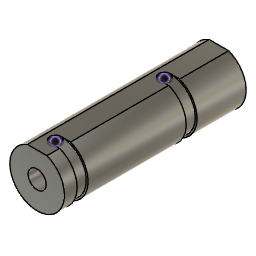
Chronograph v3 (Autodesk Fusion 360 design; units mm, degrees)
Autodesk Fusion 360 part; units mm, degrees
sketch "Sketch1" plane through (0, 0, 0) normal (0, 1, 0) x (1, 0, 0)
  circle A0 centre (0, 0) radius 7.25
  circle A1 centre (0, 0) radius 2.25
  dimension "d1" = 14.5
  dimension "d2" = 4.5
  constraint coincident A0.centre A1.centre
  measures "d1" diameter of A0
  measures "d2" diameter of A1
extrude "Extrude1" add sketch "Sketch1" along normal blind 20 makes body 1
sketch "Sketch2" plane through (0, 0, 0) normal (0, -1, 0) x (1, 0, 0)
  circle A0 centre (0, 0) radius 2.25
  circle A1 centre (0, 0) radius 7.25
  circle A2 centre (0, 0) radius 7.25
  circle A3 centre (0, 0) radius 7.35
  circle A4 centre (0, 0) radius 15
  circle A5 centre (0, 0) radius 5
  dimension "d5" = 0.1
  dimension "d6" = 30
  dimension "d7" = 10
  constraint concentric A2 A4
  constraint coincident A0.centre A1.centre
  measures "d6" diameter of A4
  measures "d7" diameter of A5
extrude "Extrude2" add sketch "Sketch2" against normal blind 20 separate body contours A4 makes body 2
extrude "Extrude3" add sketch "Sketch2" along normal blind 80 contours A1 A2 | A3 | A4 bodies 2
sketch "Sketch3" plane through (0, 0, 0) normal (0, 0, 1) x (1, 0, 0)
  line L0 (-27.4717, -70) -> (30.3284, -70) construction
  line L1 (-28.0905, -10) -> (-26.9766, -10)
  line L2 (-26.9766, -10) -> (39.3636, -10) construction
  line L3 (-15, -80) -> (15, -80)
  circle A0 through (-15, -80, 0) (7.5, -80, 12.9904) (7.5, -80, -12.9904)
  line L4 (0, -70) -> (0, -10) construction
  circle A1 centre (0, -10) radius 2.5
  circle A2 centre (0, -70) radius 2.5
  dimension "d12" = 10
  dimension "d13" = 60
  dimension "d14" = 5
  dimension "d15" = 5
  constraint horizontal L0
  constraint horizontal L1
  constraint parallel L1 L2
  constraint coincident L2 L4.end
  constraint coincident L0 L4.start
  constraint coincident L4.end A1.centre
  constraint coincident L4.start A2.centre
  measures "d12" distance of L0 L3
  measures "d13" distance of L0 L2
  measures "d14" diameter of A1
  measures "d15" diameter of A2
extrude "Extrude4" cut sketch "Sketch3" along normal mid plane 32 bodies 2
ref_plane "WorkPlane1" through (0, 0, 13) normal (0, 0, 1) x (1, 0, 0)
ref_plane "WorkPlane2" through (0, 0, -13) normal (0, 0, 1) x (1, 0, 0)
sketch "Sketch4" plane through (0, 0, 13) normal (0, 0, 1) x (1, 0, 0)
  circle A0 centre (0, -10) radius 2.5
  circle A1 centre (0, -10) radius 3
  circle A2 centre (0, -70) radius 2.5
  circle A3 centre (0, -70) radius 3
  dimension "d20" = 6
  dimension "d21" = 6
  constraint concentric A0 A1
  constraint concentric A2 A3
  measures "d20" diameter of A1
  measures "d21" diameter of A3
extrude "Extrude5" cut sketch "Sketch4" along normal blind 9 contours A0 | A1 | A2 | A3 bodies 2
sketch "Sketch5" plane through (0, 0, -13) normal (0, 0, 1) x (1, 0, 0)
  circle A0 centre (0, -10) radius 3
  circle A1 centre (0, -70) radius 3
extrude "Extrude6" cut sketch "Sketch5" against normal blind 6 bodies 2
ref_plane "WorkPlane3" through (0, -70, 14) normal (0, 0, 1) x (1, 0, 0)
sketch "Sketch6" plane through (0, 0, 14) normal (0, 0, 1) x (1, 0, 0)
  line L0 (-34.0055, 38.0437) -> (36.5157, 38.0437)
  line L1 (36.5157, 38.0437) -> (36.5157, -94.6762)
  line L2 (36.5157, -94.6762) -> (-34.0055, -94.6762)
  line L3 (-34.0055, -94.6762) -> (-34.0055, 38.0437)
  constraint horizontal L0
  constraint vertical L1
  constraint horizontal L2
  constraint vertical L3
extrude "Extrude7" cut sketch "Sketch6" along normal blind 8 bodies 2
sketch "Sketch7" plane through (0, 0, 0) normal (1, 0, 0) x (0, 1, 0)
  line L0 (-7, 14) -> (-13, 14)
  line L1 (-67, 14) -> (-73, 14)
  line L2 (-73, 14) -> (-67, 14)
  line L3 (-67, 14) -> (-67, 17.2826)
  line L4 (-67, 17.2826) -> (-73, 17.2826)
  line L5 (-73, 17.2826) -> (-73, 14)
  line L6 (-13, 14) -> (-7, 14)
  line L7 (-7, 14) -> (-7, 17.9339)
  line L8 (-7, 17.9339) -> (-13, 17.9339)
  line L9 (-13, 17.9339) -> (-13, 14)
  constraint horizontal L2
  constraint vertical L3
  constraint horizontal L4
  constraint vertical L5
  constraint coincident L1.end L2.start
  constraint horizontal L6
  constraint vertical L7
  constraint horizontal L8
  constraint vertical L9
  constraint coincident L0.end L6.start
revolve "Revolve1" cut sketch "Sketch7" angle 180 about axis through (0, 0, 0) along (0, 1, 0) bodies 2
hidden bodies 1
named bodies: "Barrel", "Chronograph"
